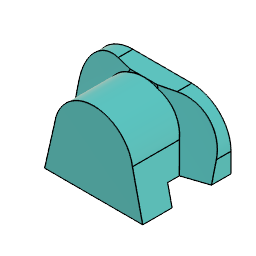
USB Port Housing (Autodesk Fusion 360 archive; units mm, degrees)
design "gasket"
Autodesk Fusion 360 part; units mm, degrees
sketch "Sketch1" plane through (0, 0, 0) normal (0, 1, 0) x (1, 0, 0)
  line L0 (-7, 0) -> (7, 0)
  line L1 (7, 0) -> (7, -6)
  line L2 (7, -6) -> (-7, -6)
  line L3 (-7, -6) -> (-7, 0)
  dimension "d1" = 14
  dimension "d2" = 6
  constraint horizontal L0
  constraint vertical L1
  constraint horizontal L2
  constraint vertical L3
  measures "d1" distance of L0.start L0.end
  measures "d2" distance of L0.start L2.end
ref_plane "WorkPlane1" through (0, -7, 3) normal (0, 1, 0) x (1, 0, 0)
sketch "Sketch4" plane through (0, -7, 0) normal (0, 1, 0) x (1, 0, 0)
  line L0 (-5, 2) -> (5, 2)
  circle A0 centre (0, -2) radius 4 construction
  line L1 (-5, 2) -> (-3.954, -2.6048)
  line L2 (5, 2) -> (3.954, -2.6048)
  line L3 (-3.954, -2.6048) -> (3.954, -2.6048) construction
  arc A1 (-3.954, -2.6048) -> (3.954, -2.6048) centre (0, -2) ccw
  dimension "d6" = 8
  constraint horizontal L0
  constraint coincident A0 L1.end
  constraint coincident A0 L2.end
  constraint horizontal L3
  measures "d6" diameter of A0
extrude "Extrude1" add sketch "Sketch4" along normal up to surface (7 mm away)
sketch "Sketch5" plane through (0, 0, 0) normal (0, 0, 1) x (1, 0, 0)
  line L0 (7, 0) -> (-7, 0)
  line L1 (-7, 0) -> (-7, -2)
  line L2 (-7, -2) -> (7, -2) construction
  line L3 (7, -2) -> (7, 0)
  line L4 (7, -2) -> (4, -3)
  line L5 (4, -3) -> (-4, -3)
  line L6 (-4, -3) -> (-7, -2)
  dimension "d9" = 14
  dimension "d10" = 2
  constraint horizontal L0
  constraint vertical L1
  constraint horizontal L2
  constraint vertical L3
  constraint perpendicular L3 L5
  measures "d9" distance of L0.start L0.end
  measures "d10" distance of L0.start L2.end
ref_plane "WorkPlane2" through (0, 0, 6) normal (0, 0, 1) x (1, 0, 0)
sketch "Sketch6" plane through (0, 0, 6) normal (0, 0, 1) x (1, 0, 0)
  line L0 (7, 0) -> (-7, 0)
  line L1 (-7, 0) -> (-7, -0.5)
  line L2 (-7, -0.5) -> (7, -0.5) construction
  line L3 (7, -0.5) -> (7, 0)
  line L4 (-1.3797, -1.9) -> (-7, -0.5)
  line L5 (0, 1.75) -> (0, 22.5)
  line L6 (-1.3797, -1.9) -> (1.3797, -1.9)
  line L7 (1.3797, -1.9) -> (7, -0.5)
  point P0 (1.3797, -1.9)
  dimension "d12" = 14
  dimension "d13" = 0.5
  dimension "d26" = 1.9
  constraint horizontal L0
  constraint vertical L1
  constraint horizontal L2
  constraint vertical L3
  constraint symmetric L4.start L5 P0
  constraint coincident P0 L6.end
  measures "d12" distance of L0.start L0.end
  measures "d13" distance of L0.start L2.end
  measures "d26" distance of L0 L6
loft "Loft1" add profiles "Sketch6", "Sketch5" section 1 section 2
fillet "Fillet1" radius 4 2 edges at (7, -0.25, 6) (-7, -0.25, 6)
sketch "Sketch7" plane through (0, 0, 0) normal (0, 0, 1) x (1, 0, 0)
  circle A0 centre (0, 13) radius 17.5
  line L0 (-7.0413, -3.0209) -> (7, -3.0209)
  line L1 (7, -3.0209) -> (7, -4)
  line L2 (7, -4) -> (-7.0413, -4)
  line L3 (-7.0413, -4) -> (-7.0413, -3.0209)
  dimension "d16" = 35
  constraint horizontal L0
  constraint vertical L1
  constraint horizontal L2
  constraint vertical L3
  constraint coincident A0 L0.start
  measures "d16" diameter of A0
extrude "Extrude2" cut sketch "Sketch7" against normal blind 5
sketch "Sketch8" plane through (0, 0, 0) normal (0, 1, 0) x (1, 0, 0)
  circle A0 centre (0, -2) radius 2.5
  circle A1 centre (0, -2) radius 1.75
  dimension "d19" = 5
  dimension "d20" = 3.5
  constraint concentric A0 A1
  measures "d19" diameter of A0
  measures "d20" diameter of A1
extrude "Extrude3" add sketch "Sketch8" against normal up to surface (7 mm away)
